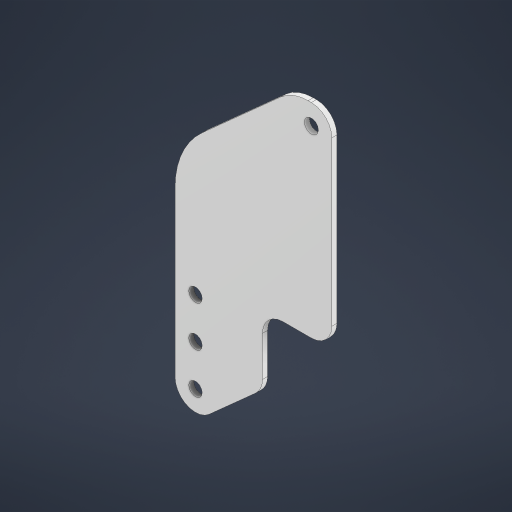
# Autodesk Inventor part: sled
Saved by Autodesk Inventor 2024 (Build 280153000, 153)
## iProperties
Created: 2024-01-16
Part Number: sled
Material: Acetal Resin, White
Document SubType Name: Modeling
Designer: avere
Density: 1.425 g/cm^3
Appearance: Smooth - White
d1: 0.500 in
d5: 0.165 in
d6: 0.165 in
Author: avere
Autodesk Inventor part; units mm, degrees
ref_plane "YZ Plane" through (0, 0, 0) normal (1, 0, 0) x (0, 1, 0)
ref_plane "XZ Plane" through (0, 0, 0) normal (0, 1, 0) x (-1, 0, 0)
ref_plane "XY Plane" through (0, 0, 0) normal (0, 0, 1) x (1, 0, 0)
sketch "main" plane through (0, 0, 0) normal (0, 0, 1) x (1, 0, 0)
  line L0 (-27.3481, 7.6574) -> (-27.3481, 8.0441)
  circle A0 centre (-20.9981, -17.7426) radius 2.0955
  line L1 (-27.3481, -43.1426) -> (-27.3481, 8.0441)
  line L2 (-16.7649, -47.8757) -> (-2.2574, -34.9005)
  circle A1 centre (-20.9981, -43.1426) radius 2.0955
  arc A2 (-27.3481, -43.1426) -> (-20.9981, -49.4926) centre (-20.9981, -43.1426) ccw
  arc A3 (-27.3481, -43.1426) -> (-16.7649, -47.8757) centre (-20.9981, -43.1426) ccw
  arc A4 (21.4453, 45.7574) -> (15.0953, 52.1074) centre (15.0953, 45.7574) ccw
  arc A5 (-18.881, 26.9766) -> (-27.3481, 8.0441) centre (-1.9481, 8.0441) ccw
  line L3 (21.4453, 45.7574) -> (21.4453, -5.0426)
  line L4 (5.602, 48.8737) -> (-18.881, 26.9766)
  circle A6 centre (15.0953, 45.7574) radius 2.1844
  line L5 (15.0953, 52.1074) -> (14.0684, 52.1074)
  arc A7 (14.0684, 52.1074) -> (5.602, 48.8737) centre (14.0684, 39.4074) ccw
  circle A8 centre (15.0953, -5.0426) radius 2.1844
  arc A9 (15.0953, -11.3926) -> (21.4453, -5.0426) centre (15.0953, -5.0426) ccw
  line L6 (15.0953, -11.3926) -> (6.2094, -11.3926)
  line L7 (-0.1406, -17.7426) -> (-0.1406, -30.1674)
  arc A10 (6.2094, -11.3926) -> (-0.1406, -17.7426) centre (6.2094, -17.7426) ccw
  arc A11 (-2.2574, -34.9005) -> (-0.1406, -30.1674) centre (-6.4906, -30.1674) ccw
  point P0 (-2.0277, 1.4023)
  point P1 (-0.1406, -33.0073)
  point P2 (9.2176, 52.1074)
  dimension "d1" = 12.7
  dimension "d5" = 4.191
  dimension "d6" = 4.191
  dimension "d8" = 4.3688
  dimension "d9" = 6.35
  measures "d1" radius of A7
  measures "d5" diameter of A0
  measures "d6" diameter of A1
  measures "d8" diameter of A8
  measures "d9" radius of A10
sketch "Sketch1" plane through (0, 0, 0) normal (0, 0, 1) x (1, 0, 0)
  circle A0 centre (-36.0934, -76.2) radius 2.0955
  line L0 (-42.4434, -38.1) -> (-42.4434, -37.7133)
  circle A1 centre (-36.0934, -63.5) radius 2.0955
  line L1 (-42.4434, -88.9) -> (-42.4434, -37.7133)
  line L2 (-31.8602, -93.6331) -> (-17.3527, -80.6579)
  circle A2 centre (-36.0934, -88.9) radius 2.0955
  arc A3 (-42.4434, -88.9) -> (-36.0934, -95.25) centre (-36.0934, -88.9) ccw
  arc A4 (-42.4434, -88.9) -> (-31.8602, -93.6331) centre (-36.0934, -88.9) ccw
  arc A5 (6.35, 0) -> (0, 6.35) centre (0, 0) ccw
  arc A6 (-33.9762, -18.7808) -> (-42.4434, -37.7133) centre (-17.0434, -37.7133) ccw
  line L3 (6.35, 0) -> (6.35, -50.8)
  line L4 (-9.4933, 3.1162) -> (-33.9762, -18.7808)
  circle A7 centre (0, 0) radius 2.1844
  line L5 (0, 6.35) -> (-1.0269, 6.35)
  arc A8 (-1.0269, 6.35) -> (-9.4933, 3.1162) centre (-1.0269, -6.35) ccw
  circle A9 centre (0, -50.8) radius 2.1844
  arc A10 (0, -57.15) -> (6.35, -50.8) centre (0, -50.8) ccw
  line L6 (0, -57.15) -> (-8.8859, -57.15)
  line L7 (-15.2359, -63.5) -> (-15.2359, -75.9248)
  arc A11 (-8.8859, -57.15) -> (-15.2359, -63.5) centre (-8.8859, -63.5) ccw
  arc A12 (-17.3527, -80.6579) -> (-15.2359, -75.9248) centre (-21.5859, -75.9248) ccw
  point P0 (-42.4434, -38.1)
  dimension "d4" = 4.191
  constraints: 1 centre point, 1 other
  measures "d4" diameter of A0
extrude "Extrusion1" add sketch "Sketch1" along normal blind 1.5875 contours L0 A6 L4 A8 L5 A5 L3 A10 L6 A11 L7 A12 L2 A4 A3 L1 | A9
body "Solid1"
